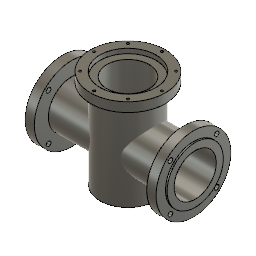
Task2d v0 (Autodesk Fusion 360 design; units mm, degrees)
Autodesk Fusion 360 part; units mm, degrees
sketch "Sketch1" plane through (0, 0, 0) normal (0, 1, 0) x (1, 0, 0)
  circle A0 centre (0, 0) radius 6
extrude "Extrude1" add sketch "Sketch1" along normal blind 20 makes body 1
sketch "Sketch2" plane through (0, 20, 0) normal (0, 1, 0) x (-1, 0, 0)
  circle A0 centre (0, 0) radius 6
  circle A1 centre (0, 0) radius 4.5
  dimension "d5" = 9
  constraint concentric A0 A1
  measures "d5" diameter of A1
extrude "Extrude2" cut sketch "Sketch2" against normal blind 19 contours A1 bodies 1
sketch "Sketch4" plane through (0, 20, 0) normal (0, 1, 0) x (-1, 0, 0)
  circle A0 centre (0, 0) radius 4.5
  circle A1 centre (0, 0) radius 6
  circle A2 centre (0, 0) radius 8
  dimension "d13" = 16
  constraint coincident A0.centre A1.centre
  measures "d13" diameter of A2
extrude "Extrude4" add sketch "Sketch4" along normal mid plane 2 contours A2 bodies 1
sketch "Sketch5" plane through (0, 21, 0) normal (0, 1, 0) x (-1, 0, 0)
  circle A0 centre (0, 0) radius 6
  circle A1 centre (0, 0) radius 8
  circle A2 centre (-0.03, -7.2499) radius 0.25
  circle A3 centre (-0.03, 7.2499) radius 0.25
  circle A4 centre (7.25, 0) radius 0.25
  circle A5 centre (-7.25, 0) radius 0.25
  line L0 (0, 0) -> (7.25, 0) construction
  circle A6 centre (-5.1265, 5.1265) radius 0.25
  circle A7 centre (5.1265, 5.1265) radius 0.25
  circle A8 centre (-5.1265, -5.1265) radius 0.25
  circle A9 centre (5.1265, -5.1265) radius 0.25
  dimension "d17" = 0.5
  dimension "d18" = 0.5
  dimension "d19" = 0.5
  dimension "d20" = 0.5
  dimension "d22" = 0.5
  dimension "d23" = 0.5
  dimension "d24" = 0.5
  dimension "d25" = 0.5
  constraint horizontal L0
  measures "d17" diameter of A2
  measures "d18" diameter of A3
  measures "d19" diameter of A4
  measures "d20" diameter of A5
  measures "d22" diameter of A6
  measures "d23" diameter of A7
  measures "d24" diameter of A8
  measures "d25" diameter of A9
extrude "Extrude5" cut sketch "Sketch5" against normal through all contours A2 | A3 | A4 | A5 | A6 | A7 | A8 | A9 bodies 1
sketch "Sketch6" plane through (0, 0, 0) normal (1, 0, 0) x (0, 0, -1)
fillet "Fillet1" radius 0.5 1 edges at (-5.594, 19, -2.1697) on bodies 1
sketch "Sketch7" plane through (0, 0, 0) normal (1, 0, 0) x (0, 0, -1)
sketch "Sketch8" plane through (0, 0, 0) normal (1, 0, 0) x (0, 0, -1)
  circle A0 centre (0, 9) radius 5
  dimension "d33" = 10
  measures "d33" diameter of A0
extrude "Extrude6" add sketch "Sketch8" along normal blind 12 separate body makes body 2
sketch "Sketch9" plane through (12, 0, 0) normal (1, 0, 0) x (0, 0, -1)
  circle A0 centre (0, 9) radius 5
  circle A1 centre (0, 9) radius 4.5
  dimension "d34" = 9
  constraint concentric A0 A1
  measures "d34" diameter of A1
extrude "Extrude7" cut sketch "Sketch9" against normal through all contours A1 bodies 1 2
sketch "Sketch10" plane through (12, 0, 0) normal (1, 0, 0) x (0, 0, -1)
  circle A0 centre (0, 9) radius 4.5
  circle A1 centre (0, 9) radius 5
  circle A2 centre (0, 9) radius 8
  dimension "d36" = 16
  constraint concentric A0 A2
  measures "d36" diameter of A2
extrude "Extrude8" add sketch "Sketch10" along normal blind 2 contours A2 bodies 2
sketch "Sketch11" plane through (14, 0, 0) normal (1, 0, 0) x (0, 0, -1)
  circle A0 centre (0, 9) radius 5
  circle A1 centre (0, 9) radius 8
  circle A2 centre (0, 9) radius 6
  dimension "d40" = 12
  constraint concentric A0 A2
  measures "d40" diameter of A2
extrude "Extrude9" add sketch "Sketch11" along normal blind 0.35 contours A2 bodies 2
extrude "Extrude10" add 1 faces at (12, 8.528, -4.798) along direction (1, 0, 0) blind 2.35 on bodies 2 bodies 2
mirror "Mirror2" about plane through (0, 0, 0) normal (-1, 0, 0) of bodies 2 1 makes body 3 at (-3.3389, 9.2106, 4.9852) makes body 4 at (-8, 8.7508, -4.9938)
sketch "Sketch13" plane through (0, 20, 0) normal (0, 1, 0) x (-1, 0, 0)
  circle A0 centre (0, 0) radius 4.5
  circle A1 centre (0, 0) radius 6
  circle A2 centre (0, 0) radius 4.5
  constraint concentric A0 A2
extrude "Extrude12" cut sketch "Sketch13" against normal blind 19 contours A0 A2 bodies 2 4
sketch "Sketch14" plane through (-14, 0, 0) normal (-1, 0, 0) x (0, 0, 1)
  circle A0 centre (0, 9) radius 6
  circle A1 centre (0, 9) radius 8
  line L0 (0, 9) -> (7, 9) construction
  circle A2 centre (4.9497, 13.9497) radius 0.5
  circle A3 centre (4.9497, 4.0503) radius 0.5
  circle A4 centre (-4.9497, 4.0503) radius 0.5
  circle A5 centre (-4.9497, 13.9497) radius 0.5
  constraint horizontal L0
extrude "Extrude13" cut sketch "Sketch14" against normal blind 2 contours A2 | A3 | A4 | A5 bodies 4
sketch "Sketch15" plane through (14, 0, 0) normal (1, 0, 0) x (0, 0, -1)
  circle A0 centre (0, 9) radius 6
  circle A1 centre (0, 9) radius 8
  circle A2 centre (4.9497, 13.9497) radius 0.5
  circle A3 centre (4.9497, 4.0503) radius 0.5
  circle A4 centre (-4.9497, 4.0503) radius 0.5
  circle A5 centre (-4.9497, 13.9497) radius 0.5
extrude "Extrude14" cut sketch "Sketch15" against normal blind 2 contours A2 | A3 | A4 | A5 bodies 2
